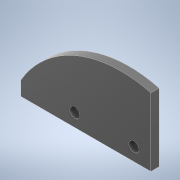
# Autodesk Inventor part: PCB-EncoderSensor
Saved by Autodesk Inventor 2022 (Build 260153000, 153)
## iProperties
Created: 2024-07-01
Part Number: PCB-EncoderSensor
Material: 一般
Document SubType Name: Modeling
Designer: yamashita1
Density: 1 g/cm^3
Appearance: 滑らか - 黒
Author: yamashita1
Autodesk Inventor part; units mm, degrees
ref_plane "YZ Plane" through (0, 0, 0) normal (1, 0, 0) x (0, 1, 0)
ref_plane "XZ Plane" through (0, 0, 0) normal (0, 1, 0) x (-1, 0, 0)
ref_plane "XY Plane" through (0, 0, 0) normal (0, 0, 1) x (1, 0, 0)
derived "FS90-Mount2.ipt"
sketch "スケッチ1" plane through (0, 0, 0) normal (0, 0, 1) x (1, 0, 0)
  circle A0 centre (0, 0) radius 23.5 construction
  circle A1 centre (0, 0) radius 22.5 construction
  line L0 (0, 0) -> (0, 27.4619) construction
  line L1 (-22.5662, 22.5662) -> (0, 0) construction
  line L2 (-16.0851, 11) -> (6.5472, 11) construction
  line L3 (2.5, 14.8525) -> (2.5, -3.8192) construction
  line L4 (-9, -3.8192) -> (-9, 14.8525) construction
  line L5 (0, 0) -> (6.8883, 25.7074) construction
  line L6 (-24.0912, 13.9091) -> (0, 0) construction
  line L7 (-19.4856, 8.5) -> (5.8234, 8.5)
  line L8 (5.8234, 8.5) -> (5.8234, 21.7333)
  line L9 (-19.4856, 11.25) -> (-19.4856, 8.5)
  arc A2 (5.8234, 21.7333) -> (-19.4856, 11.25) centre (0, 0) ccw
  circle A3 centre (2.5, 11) radius 1
  circle A4 centre (-9, 11) radius 1
  dimension "d1" = 47
  dimension "d2" = 1
  dimension "d3" = 45
  dimension "d4" = 11
  dimension "d5" = 2.5
  dimension "d6" = 9
  dimension "d7" = 15
  dimension "d8" = 15
  dimension "d9" = 8.5
  dimension "d10" = 2
  constraints: 22 end point, 6 point on line, 5 centre point, 4 point on circle, 2 coincident, 2 horizontal, 2 perpendicular, 2 vertical, 1 concentric, 1 equal radius
  measures "d1" diameter of A0
  measures "d2" radial gap between concentric circles of A0 A1
  measures "d3" angle of L1 L0
  measures "d4" distance from line of point (0, 0) L2
  measures "d5" distance between parallel lines of L0 L3
  measures "d6" distance between parallel lines of L0 L4
  measures "d7" angle of L0 L5
  measures "d8" angle of L1 L6
  measures "d9" distance from line of point (0, 0) L7
  measures "d10" diameter of A3
extrude "押し出し1" add sketch "スケッチ1" along normal blind 1.6
equation "\"d1\" = WHEEL_DIA"
equation "\"d2\" = WHEEL_CLEARANCE"
equation "\"d3\" = SENSOR_ANGLE"
equation "\"d4\" = H_OFFSET"
equation "\"d5\" = X_OFFSET1"
equation "\"d6\" = X_OFFSET2"
equation "\"d8\" = d7"
equation "\"WHEEL_DIA\" = 47"
equation "\"WHEEL_CLEARANCE\" = 1"
equation "\"SENSOR_ANGLE\" = 45deg"
equation "\"X_OFFSET1\" = 2.5"
equation "\"X_OFFSET2\" = 9"
equation "\"H_OFFSET\" = 11"
